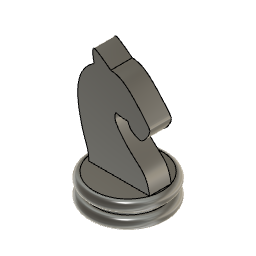
knight chess piece (Autodesk Fusion 360 design; units mm, degrees)
Autodesk Fusion 360 part; units mm, degrees
sketch "Sketch1" plane through (0, 0, 0) normal (0, 1, 0) x (1, 0, 0)
  line L0 (15, -25) -> (-15, -25) construction
  line L1 (-15, -25) -> (-15, 25) construction
  line L2 (-15, 25) -> (15, 25) construction
  line L3 (15, 25) -> (15, -25) construction
  line L4 (15, -25) -> (-15, 25) construction
  line L5 (-15, -25) -> (15, 25) construction
  line L6 (0, 22.9999) -> (12.6, 22.9999)
  circle A0 centre (12.6206, 15.5541) radius 2
  circle A1 centre (12.6, 20.9999) radius 2
  line L7 (12.6206, 13.5541) -> (0, 13.5541)
  line L8 (0, 13.5541) -> (0, 22.9999)
  line L9 (11.9848, 17.4504) -> (11.9848, 19.0969)
  line L10 (12.6, 20.9999) -> (12.6, 22.9999) construction
  dimension "d1" = 30
  dimension "d2" = 50
  dimension "d3" = 4
  dimension "d4" = 12.6206
  dimension "d5" = 9.4458
  dimension "d6" = 12.6
  dimension "d7" = 1.6465
  dimension "d8" = 13.5541
  constraint horizontal L0
  constraint perpendicular L0 L1
  constraint parallel L0 L2
  constraint parallel L1 L3
  constraint coincident L4 origin
  constraint coincident L5 origin
  constraint perpendicular L3 L6
  constraint coincident A0 L7.start
  constraint tangent A0 L7
  constraint horizontal L7
  constraint perpendicular L6 L8
  constraint coincident A0 L9.start
  constraint coincident A1 L9.end
  constraint vertical L9
  constraint equal A0 A1
  constraint coincident A1.centre L10.start
  constraint coincident A1 L6.end
  constraint parallel L3 L10
  constraint coincident L6.end L10.end
  constraint vertical origin L7.end
  measures "d1" distance of L1.end L2.end
  measures "d2" distance of L0.end L1.end
  measures "d3" diameter of A0
  measures "d4" distance of L7.start L7.end
  measures "d5" distance of L6.start L7.end
  measures "d6" distance of L6.start L6.end
  measures "d7" distance of L9.start L9.end
  measures "d8" distance of origin L7.end
revolve "Revolve1" add sketch "Sketch1" angle 360 about axis through (0, 0, 1.75) along (0, 0, 1)
sketch "Sketch2" plane through (0, 0, 0) normal (0, 1, 0) x (1, 0, 0)
  spline S0 degree 5 poles (-10.6015, 13.5619) (-10.5938, 13.5095) (-10.5811, 13.3936) (-10.5707, 13.1868) (-10.5743, 12.845) (-10.6084, 12.3126) (-10.6742, 11.693) (-10.775, 11.0177) (-10.9135, 10.3197) (-11.0909, 9.6246) (-11.3043, 8.9384) (-11.5475, 8.2466) (-11.8127, 7.5262) (-12.0914, 6.7523) (-12.3765, 5.9084) (-12.6632, 4.9911) (-12.9476, 4.0054) (-13.2266, 2.9623) (-13.4969, 1.8747) (-13.7547, 0.7551) (-13.9947, -0.3884) (-14.2106, -1.551) (-14.395, -2.73) (-14.54, -3.9235) (-14.6376, -5.1296) (-14.6795, -6.3451) (-14.6576, -7.564) (-14.5645, -8.7781) (-14.393, -9.9777) (-14.137, -11.1523) (-13.791, -12.2917) (-13.3507, -13.3867) (-12.8129, -14.43) (-12.1758, -15.4168) (-11.4387, -16.3439) (-10.6012, -17.2099) (-9.8512, -17.8533) (-9.2439, -18.308) (-8.819, -18.5988) (-8.6016, -18.7411) knots 0 0 0 0 0 0 0.028571 0.057143 0.085714 0.114286 0.142857 0.171429 0.2 0.228571 0.257143 0.285714 0.314286 0.342857 0.371429 0.4 0.428571 0.457143 0.485714 0.514286 0.542857 0.571429 0.6 0.628571 0.657143 0.685714 0.714286 0.742857 0.771429 0.8 0.828571 0.857143 0.885714 0.914286 0.942857 0.971429 1 1 1 1 1 1
  line L0 (-10.6015, 13.5619) -> (12, 13.5619)
  spline S1 degree 5 poles (12, 13.5619) (11.9688, 13.3792) (11.9044, 13.0189) (11.8025, 12.4934) (11.6558, 11.8232) (11.4533, 11.0358) (11.2289, 10.2973) (10.9775, 9.6046) (10.6905, 8.9521) (10.3547, 8.331) (9.9555, 7.7299) (9.4795, 7.1358) (8.9175, 6.5354) (8.268, 5.9155) (7.539, 5.2642) (6.7455, 4.5719) (5.9079, 3.8326) (5.0493, 3.0446) (4.1937, 2.2121) (3.3643, 1.3457) (2.5806, 0.4648) (1.8588, -0.4058) (1.2113, -1.2402) (0.6472, -2.0151) (0.1724, -2.714) (-0.211, -3.331) (-0.5042, -3.8758) (-0.7111, -4.3726) (-0.8373, -4.8506) (-0.888, -5.3377) (-0.8669, -5.852) (-0.7945, -6.292) (-0.7092, -6.6393) (-0.6387, -6.8785) (-0.6, -7) knots 0 0 0 0 0 0 0.033333 0.066667 0.1 0.133333 0.166667 0.2 0.233333 0.266667 0.3 0.333333 0.366667 0.4 0.433333 0.466667 0.5 0.533333 0.566667 0.6 0.633333 0.666667 0.7 0.733333 0.766667 0.8 0.833333 0.866667 0.9 0.933333 0.966667 1 1 1 1 1 1
  spline S2 degree 5 poles (-0.6, -7) (-0.5664, -6.9934) (-0.4984, -6.98) (-0.3945, -6.9592) (-0.2519, -6.9303) (-0.0669, -6.8921) (0.125, -6.852) (0.3236, -6.8104) (0.5287, -6.7679) (0.74, -6.7254) (0.957, -6.6839) (1.1792, -6.6445) (1.4065, -6.6083) (1.6387, -6.5759) (1.8762, -6.5479) (2.1192, -6.5246) (2.3682, -6.5063) (2.6235, -6.4929) (2.8853, -6.4844) (3.1538, -6.4809) (3.4289, -6.4822) (3.6541, -6.487) (3.826, -6.4927) (3.9418, -6.4974) (4, -6.5) knots 0 0 0 0 0 0 0.05 0.1 0.15 0.2 0.25 0.3 0.35 0.4 0.45 0.5 0.55 0.6 0.65 0.7 0.75 0.8 0.85 0.9 0.95 1 1 1 1 1 1
  spline S3 degree 5 poles (4, -6.5) (3.9927, -6.4898) (3.9818, -6.465) (3.977, -6.4145) (3.9936, -6.3206) (4.0499, -6.1583) (4.1347, -5.9484) (4.2417, -5.6903) (4.3719, -5.3882) (4.5375, -5.0537) (4.7555, -4.7026) (5.0412, -4.3521) (5.4021, -4.0178) (5.8301, -3.7102) (6.3017, -3.4343) (6.7864, -3.1922) (7.2527, -2.985) (7.6753, -2.8146) (8.0411, -2.686) (8.3576, -2.6096) (8.646, -2.5981) (8.9309, -2.6625) (9.2316, -2.8085) (9.5525, -3.0322) (9.8871, -3.3226) (10.2227, -3.665) (10.545, -4.043) (10.8421, -4.4414) (11.1089, -4.849) (11.3441, -5.2572) (11.5486, -5.6597) (11.7229, -6.0513) (11.865, -6.4278) (11.9685, -6.7847) (12.0242, -7.1184) (12.0246, -7.4273) (11.9657, -7.7127) (11.852, -7.9807) (11.6933, -8.2407) (11.5006, -8.504) (11.2822, -8.7825) (11.0391, -9.0867) (10.768, -9.4257) (10.4628, -9.8064) (10.1173, -10.233) (9.727, -10.7069) (9.2913, -11.2253) (8.8134, -11.7828) (8.2988, -12.3713) (7.755, -12.9812) (7.1903, -13.6019) (6.6136, -14.2223) (6.0327, -14.832) (5.4543, -15.4213) (4.883, -15.9826) (4.3205, -16.5103) (3.7668, -17.0002) (3.2204, -17.4499) (2.6787, -17.858) (2.1383, -18.2238) (1.5957, -18.5474) (1.0478, -18.829) (0.492, -19.0691) (-0.0735, -19.2679) (-0.6499, -19.4257) (-1.2378, -19.5426) (-1.7177, -19.6035) (-2.083, -19.6308) (-2.329, -19.6409) (-2.4525, -19.644) knots 0 0 0 0 0 0 0.01538462 0.03076923 0.04615385 0.06153846 0.07692308 0.09230769 0.10769231 0.12307692 0.13846154 0.15384615 0.16923077 0.18461538 0.2 0.21538462 0.23076923 0.24615385 0.26153846 0.27692308 0.29230769 0.30769231 0.32307692 0.33846154 0.35384615 0.36923077 0.38461538 0.4 0.41538462 0.43076923 0.44615385 0.46153846 0.47692308 0.49230769 0.50769231 0.52307692 0.53846154 0.55384615 0.56923077 0.58461538 0.6 0.61538462 0.63076923 0.64615385 0.66153846 0.67692308 0.69230769 0.70769231 0.72307692 0.73846154 0.75384615 0.76923077 0.78461538 0.8 0.81538462 0.83076923 0.84615385 0.86153846 0.87692308 0.89230769 0.90769231 0.92307692 0.93846154 0.95384615 0.96923077 0.98461538 1 1 1 1 1 1
  spline S4 degree 5 poles (-2.4525, -19.644) (-2.5627, -19.7317) (-2.7818, -19.9052) (-3.1065, -20.1601) (-3.5315, -20.4889) (-4.0494, -20.8814) (-4.5533, -21.255) (-5.0424, -21.6091) (-5.5149, -21.9428) (-5.9687, -22.2548) (-6.4007, -22.5437) (-6.8069, -22.8076) (-7.1827, -23.0438) (-7.5239, -23.2492) (-7.8276, -23.419) (-8.0927, -23.5474) (-8.3213, -23.6262) (-8.5187, -23.6461) (-8.6903, -23.5998) (-8.8393, -23.4853) (-8.9644, -23.3086) (-9.0614, -23.0814) (-9.1261, -22.8163) (-9.157, -22.5231) (-9.1567, -22.2061) (-9.1301, -21.8664) (-9.083, -21.5028) (-9.0215, -21.1133) (-8.9498, -20.6966) (-8.8707, -20.2519) (-8.786, -19.7789) (-8.7145, -19.3779) (-8.6588, -19.0644) (-8.6208, -18.8498) (-8.6016, -18.7411) knots 0 0 0 0 0 0 0.033333 0.066667 0.1 0.133333 0.166667 0.2 0.233333 0.266667 0.3 0.333333 0.366667 0.4 0.433333 0.466667 0.5 0.533333 0.566667 0.6 0.633333 0.666667 0.7 0.733333 0.766667 0.8 0.833333 0.866667 0.9 0.933333 0.966667 1 1 1 1 1 1
  point P0 (-10.6015, 12.475)
  point P1 (-11, 10)
  point P2 (-12, 7)
  point P3 (-13.5145, 1.7798)
  point P4 (-14.6449, -5.5677)
  point P5 (-13.471, -13.0457)
  point P6 (10.9423, 9.5498)
  point P7 (9.0148, 6.6521)
  point P8 (4, 2)
  point P9 (0, -3)
  point P10 (-0.8414, -4.997)
  point P11 (0.2315, -6.8297)
  point P12 (1.268, -6.6309)
  point P13 (2.5, -6.5)
  point P14 (4, -6.3186)
  point P15 (4.2354, -5.708)
  point P16 (5.2293, -4.1888)
  point P17 (7.7321, -2.7987)
  point P18 (8.9416, -2.6853)
  point P19 (10.5, -4)
  point P20 (11.7385, -6.1058)
  point P21 (12, -7.5)
  point P22 (11.5, -8.5)
  point P23 (10.0755, -10.2823)
  point P24 (5.729, -15.139)
  point P25 (1.4077, -18.6378)
  point P26 (-6.1247, -22.3581)
  point P27 (-8.0029, -23.4997)
  point P28 (-8.7026, -23.5733)
  point P29 (-9.1, -22.9)
  point P30 (-9.0708, -21.4374)
  constraint horizontal L0
extrude "Extrude1" add sketch "Sketch2" along normal mid plane 8
